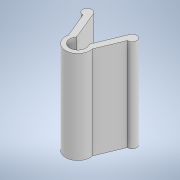
# Autodesk Inventor part: 20_Rect_Aperture_door_test
Saved by Autodesk Inventor 2022 (Build 260153000, 153)
## iProperties
Created: 2022-02-03
Part Number: 20_Rect_Aperture_door_test
Material: Generic
Document SubType Name: Modeling
Designer: UC2
Density: 1 g/cm^3
Appearance: Default
Author: UC2
Autodesk Inventor part; units mm, degrees
ref_plane "YZ Plane" through (0, 0, 0) normal (1, 0, 0) x (0, 1, 0)
ref_plane "XZ Plane" through (0, 0, 0) normal (0, 1, 0) x (-1, 0, 0)
ref_plane "XY Plane" through (0, 0, 0) normal (0, 0, 1) x (1, 0, 0)
sketch "Sketch1" plane through (0, 0, 0) normal (0, 1, 0) x (-1, 0, 0)
  line L0 (12.25, 0) -> (-12.25, 0) construction
  line L1 (0, -4.6569) -> (0, 17.4416) construction
  circle A0 centre (7.25, 0) radius 1.5
  line L2 (5.8642, -0.574) -> (2.0373, 8.6648)
  line L3 (7.1707, 1.4979) -> (3.8797, 9.4433)
  circle A1 centre (-7.25, 0) radius 1.5
  line L4 (-5.8642, -0.574) -> (-2.0373, 8.6648)
  line L5 (-7.1707, 1.4979) -> (-3.8797, 9.4433)
  arc A2 (2.0373, 8.6648) -> (-2.0373, 8.6648) centre (0, 10.3094) ccw
  arc A3 (3.8797, 9.4433) -> (-3.8797, 9.4433) centre (0, 10.3094) ccw
  point P0 (0, 0)
  dimension "d0" = 3
  dimension "d1" = 2
  dimension "d2" = 45
  dimension "d3" = 10
  dimension "d4" = 8.6
  dimension "d5" = 14.5
  constraints: 8 end point, 8 point on circle, 5 symmetric about line, 4 centre point, 1 concentric, 1 parallel, 1 point on line, 1 tangent, 1 other
  measures "d0" diameter of A0
  measures "d1" distance between parallel lines of L2 L3
  measures "d2" angle of L4 L2
  measures "d3" distance of L2.start L2.end
  measures "d4" distance of L3.start L3.end
  measures "d5" distance of A1.centre A0.centre
extrude "Extrusion1" add sketch "Sketch1" along normal blind 30
body "Solid1"
